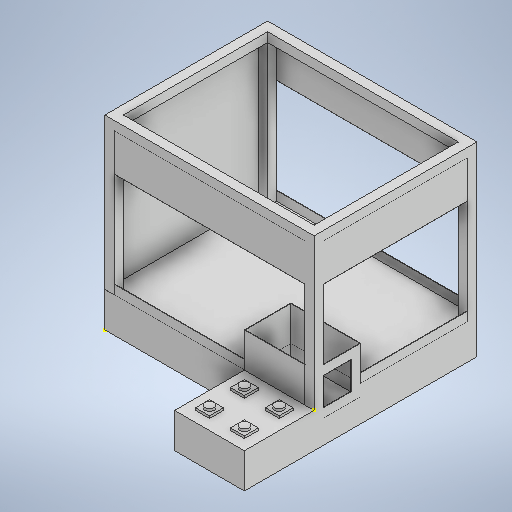
# Autodesk Inventor part: Project frame
Saved by Autodesk Inventor 2025.2 (Build 292293000, 293)
## iProperties
Created: 2025-01-26
Part Number: Project frame
Material: Generic
Document SubType Name: Modeling
Designer: Asus
Density: 1 g/cm^3
Appearance: Default
Author: Asus
Autodesk Inventor part; units mm, degrees
ref_plane "YZ Plane" through (0, 0, 0) normal (1, 0, 0) x (0, 1, 0)
ref_plane "XZ Plane" through (0, 0, 0) normal (0, 1, 0) x (-1, 0, 0)
ref_plane "XY Plane" through (0, 0, 0) normal (0, 0, 1) x (1, 0, 0)
sketch "Sketch1" plane through (0, 0, 0) normal (0, 1, 0) x (-1, 0, 0)
  line L0 (0, 0) -> (0, -350)
  line L1 (0, -350) -> (450, -350)
  line L2 (450, -350) -> (450, 0)
  line L3 (450, 0) -> (0, 0)
  dimension "d0" = 350
  dimension "d1" = 450
  constraints: 8 end point, 2 vertical, 1 horizontal, 1 perpendicular
  measures "d0" distance of L0.start L0.end
  measures "d1" distance of L0.end L1.end
extrude "Extrusion1" add sketch "Sketch1" along normal blind 75
sketch "Sketch2" plane through (0, 75, 0) normal (0, 1, 0) x (1, 0, 0)
  line L0 (-20, 350) -> (-20, 330)
  line L1 (-20, 330) -> (0, 330)
  line L2 (0, 350) -> (-450, 350) projected
  line L3 (0, 330) -> (0, 350)
  line L4 (0, 350) -> (-20, 350)
  point P0 (0, 0)
  dimension "d4" = 20
  dimension "d5" = 20
  constraints: 8 end point, 2 perpendicular, 1 collinear, 1 vertical
  measures "d4" distance of L0.start L0.end
  measures "d5" distance of L0.end L1.end
extrude "Extrusion2" add sketch "Sketch2" along normal blind 325
sketch "Sketch3" plane through (0, 75, 0) normal (0, 1, 0) x (1, 0, 0)
  point P0 (0, 0)
sketch "Sketch4" plane through (0, 75, 0) normal (0, 1, 0) x (1, 0, 0)
  line L0 (-20, 350) -> (-20, 330) projected
  line L1 (-20, 350) -> (-20, 349)
  line L2 (-20, 349) -> (-450, 349)
  line L3 (-450, 349) -> (-450, 350)
  line L4 (-450, 350) -> (-20, 350)
  line L5 (-20, 350) -> (-20, 349)
  line L6 (0, 0) -> (0, 350) projected
  line L7 (-20, 349) -> (-20, 350)
  line L8 (-20, 350) -> (-20, 349)
  dimension "d9" = 430
  dimension "d10" = 1
  dimension "d11" = 430
  dimension "d12" = 1
  constraints: 14 end point, 2 collinear, 2 perpendicular, 1 parallel, 1 point on line
  measures "d9" distance of L1.end L2.end
  measures "d10" distance of L2.end L3.end
  measures "d11" distance of L3.end L0.start
  measures "d12" distance of L0.start L1.end
extrude "Extrusion3" add sketch "Sketch4" along normal blind 20
sketch "Sketch5" plane through (0, 75, 0) normal (0, 1, 0) x (1, 0, 0)
  line L0 (-450, 350) -> (-450, 0) projected
  line L1 (-450, 350) -> (-449, 350)
  line L2 (-20, 350) -> (-450, 350) projected
  line L3 (-449, 350) -> (-449, 0)
  line L4 (-450, 0) -> (0, 0) projected
  line L5 (-449, 0) -> (-450, 0)
  line L6 (-450, 0) -> (-450, 350)
  line L7 (-20, 349) -> (-450, 349) projected
  line L8 (-449, 349) -> (-449, 350)
  line L9 (-450, 350) -> (-449, 350)
  dimension "d15" = 1
  constraints: 12 end point, 4 point on line, 3 collinear, 1 horizontal, 1 vertical
  measures "d15" distance of L0.start L1.end
extrude "Extrusion4" add sketch "Sketch5" along normal blind 325 contours L7 L3 L4 L0
sketch "Sketch6" plane through (0, 95, 0) normal (0, 1, 0) x (1, 0, 0)
  line L0 (-449, 349) -> (-449, 0) projected
  line L1 (-449, 349) -> (-449, 350)
  line L2 (-20, 350) -> (-450, 350) projected
  line L3 (-450, 350) -> (-450, 0) projected
  line L4 (-449, 350) -> (-450, 350)
  line L5 (-450, 350) -> (-450, 349)
  line L6 (-450, 349) -> (-449, 349) projected
  line L7 (-450, 349) -> (-449, 349)
  line L8 (-449, 349) -> (-449, 350)
  point P0 (0, 0)
  constraints: 10 end point, 3 collinear, 1 perpendicular, 1 point on line, 1 vertical
extrude "Extrusion5" add sketch "Sketch6" along normal blind 305
sketch "Sketch7" plane through (0, 75, 0) normal (0, 1, 0) x (1, 0, 0)
  line L0 (0, 0) -> (0, 350) projected
  line L1 (0, 0) -> (0, 20)
  line L2 (0, 20) -> (-20, 20)
  line L3 (-20, 20) -> (-20, 0)
  line L4 (-20, 0) -> (0, 0)
  dimension "d20" = 20
  dimension "d21" = 20
  constraints: 8 end point, 3 perpendicular, 1 point on line
  measures "d20" distance of L0.start L1.end
  measures "d21" distance of L1.end L2.end
extrude "Extrusion6" add sketch "Sketch7" along normal blind 325
sketch "Sketch8" plane through (0, 75, 0) normal (0, 1, 0) x (1, 0, 0)
  line L0 (0, 20) -> (-20, 20) projected
  line L1 (0, 20) -> (0, 100)
  line L2 (0, 20) -> (0, 330) projected
  line L3 (0, 100) -> (-1, 100)
  line L4 (-1, 100) -> (-1, 20)
  line L5 (-1, 20) -> (0, 20)
  point P0 (0, 0)
  dimension "d24" = 80
  dimension "d25" = 1
  dimension "d26" = 80
  constraints: 8 end point, 2 point on line, 1 collinear, 1 horizontal
  measures "d24" distance of L0.start L1.end
  measures "d25" distance of L1.end L3.end
  measures "d26" distance of L3.end L4.end
extrude "Extrusion7" add sketch "Sketch8" along normal blind 75
sketch "Sketch9" plane through (0, 75, 0) normal (0, 1, 0) x (1, 0, 0)
  line L0 (-1, 100) -> (0, 100) projected
  line L1 (-1, 100) -> (-149, 100)
  line L2 (-149, 100) -> (-149, 99)
  line L3 (-149, 99) -> (-1, 99)
  line L4 (-1, 100) -> (-1, 20) projected
  line L5 (-1, 99) -> (-1, 100)
  point P0 (0, 0)
  dimension "d29" = 148
  dimension "d32" = 1
  dimension "d33" = 148
  constraints: 8 end point, 1 horizontal, 1 perpendicular, 1 vertical
  measures "d29" distance of L0.start L1.end
  measures "d32" distance of L1.end L2.end
  measures "d33" distance of L2.end L3.end
extrude "Extrusion8" add sketch "Sketch9" along normal blind 75
sketch "Sketch10" plane through (0, 75, 0) normal (0, 1, 0) x (1, 0, 0)
  line L0 (-149, 99) -> (-149, 100) projected
  line L1 (-149, 100) -> (-150, 100)
  line L2 (-150, 100) -> (-150, 0)
  line L3 (-150, 0) -> (-149, 0)
  line L4 (-449, 0) -> (-20, 0) projected
  line L5 (-149, 0) -> (-149, 100)
  point P0 (0, 0)
  dimension "d36" = 1
  dimension "d37" = 100
  dimension "d38" = 1
  dimension "d39" = 100
  constraints: 8 end point, 1 horizontal, 1 point on line, 1 vertical
  measures "d36" distance of L0.end L1.end
  measures "d37" distance of L1.end L2.end
  measures "d38" distance of L2.end L3.end
  measures "d39" distance of L3.end L0.end
extrude "Extrusion9" add sketch "Sketch10" along normal blind 75
sketch "Sketch11" plane through (0, 75, 0) normal (0, 1, 0) x (1, 0, 0)
  line L0 (-450, 0) -> (0, 0) projected
  line L1 (-149.0001, 0) -> (-20.0001, 0)
  line L2 (-20.0001, 0) -> (-20.0001, 1)
  line L3 (-20.0001, 1) -> (-149.0001, 1)
  line L4 (-149.0001, 1) -> (-149.0001, 0)
  dimension "d42" = 129
  dimension "d43" = 1
  dimension "d44" = 129
  constraints: 8 end point, 2 perpendicular, 2 point on line
  measures "d42" distance of L1.start L1.end
  measures "d43" distance of L1.end L2.end
  measures "d44" distance of L2.end L3.end
extrude "Extrusion10" add sketch "Sketch11" along normal blind 75
sketch "Sketch12" plane through (0, 75, 0) normal (0, 1, 0) x (1, 0, 0)
  point P0 (0, 0)
sketch "Sketch13" plane through (0, 75, 0) normal (0, 1, 0) x (1, 0, 0)
  line L0 (-149, 1) -> (-149, 99) projected
  line L1 (-1, 20) -> (-1, 99) projected
  line L2 (-149, 99) -> (-1, 99)
  line L3 (-1, 99) -> (-1, 20)
  line L4 (0, 20) -> (-20, 20) projected
  line L5 (-1, 20) -> (-20, 20)
  line L6 (-20, 20) -> (-20, 1)
  line L7 (-20, 0) -> (0, 0) projected
  line L8 (-20, 1) -> (-149, 1)
  line L9 (-149, 1) -> (-149, 99)
  constraints: 12 end point, 4 perpendicular, 1 collinear, 1 horizontal
extrude "Extrusion11" cut sketch "Sketch13" against normal blind 25
sketch "Sketch14" plane through (0, 75, 0) normal (0, 1, 0) x (1, 0, 0)
  line L0 (0, 100) -> (0, 330) projected
  line L1 (0, 330) -> (0, 100)
  line L2 (0, 100) -> (-1, 100)
  line L3 (-150, 100) -> (0, 100) projected
  line L4 (0, 100) -> (1, 100) construction
  line L5 (-1, 100) -> (-1, 330)
  line L6 (-1, 330) -> (0, 330)
  point P0 (0, 0)
  dimension "d49" = 1
  dimension "d50" = 180
  dimension "d51" = 230
  dimension "d52" = 90
  constraints: 10 end point, 2 collinear, 1 horizontal, 1 perpendicular, 1 vertical
  measures "d49" distance of L0.start L2.end
  measures "d50" angle of L2 L4
  measures "d51" distance of L2.end L5.end
  measures "d52" angle of L2 L5
extrude "Extrusion12" add sketch "Sketch14" along normal blind 20
sketch "Sketch15" plane through (0, 75, 0) normal (0, 1, 0) x (1, 0, 0)
  line L0 (-449, 0) -> (-449, 350) projected
  line L1 (-150, 100) -> (-150, 0) projected
  line L2 (-449, 0) -> (-150, 0)
  line L3 (-150, 0) -> (-150, 1)
  line L4 (-150, 1) -> (-449, 1)
  line L5 (-449, 1) -> (-449, 0)
  point P0 (0, 0)
  dimension "d55" = 1
  dimension "d56" = 90
  constraints: 8 end point, 4 perpendicular
  measures "d55" distance of L1.end L3.end
  measures "d56" angle of L3 L2
extrude "Extrusion13" add sketch "Sketch15" along normal blind 20
sketch "Sketch16" plane through (0, 400, 0) normal (0, 1, 0) x (1, 0, 0)
  line L0 (-450, 350) -> (-450, 0) projected
  line L1 (-449, 0) -> (-449, 350) projected
  line L2 (-450, 350) -> (-449, 350)
  line L3 (-449, 350) -> (-449, 330)
  line L4 (-449, 330) -> (-450, 330)
  line L5 (-450, 330) -> (-450, 350)
  point P0 (0, 0)
  dimension "d59" = 20
  dimension "d60" = 20
  constraints: 8 end point, 4 perpendicular
  measures "d59" distance of L1.end L3.end
  measures "d60" distance of L4.end L0.start
extrude "Extrusion14" cut sketch "Sketch16" against normal blind 325
sketch "Sketch17" plane through (-449, 75, -349) normal (-1, 0, 0) x (0, 0, 1)
  line L0 (-1, 0) -> (-1, 20) projected
  line L1 (-1, 20) -> (-1, 0)
  line L2 (-1, 0) -> (0, 0)
  line L3 (0, 0) -> (0, 20)
  line L4 (0, 20) -> (-1, 20)
  point P0 (349, -75)
  dimension "d63" = 1
  constraints: 8 end point, 3 perpendicular, 1 vertical
  measures "d63" distance of L1.end L2.end
extrude "Extrusion15" cut sketch "Sketch17" against normal blind 19
sketch "Sketch18" plane through (0, 75, 0) normal (0, 1, 0) x (1, 0, 0)
  line L0 (-450, 350) -> (-430, 350) projected
  line L1 (-450, 350) -> (-430, 350)
  line L2 (-430, 350) -> (-430, 330)
  line L3 (-430, 330) -> (-450, 330)
  line L4 (-450, 330) -> (-450, 350)
  point P0 (0, 0)
  dimension "d66" = 20
  constraints: 8 end point, 3 perpendicular, 1 horizontal
  measures "d66" distance of L0.end L2.end
extrude "Extrusion16" add sketch "Sketch18" along normal blind 325
sketch "Sketch19" plane through (0, 400, 0) normal (0, 1, 0) x (1, 0, 0)
  line L0 (-449, 0) -> (-449, 1) projected
  line L1 (-450, 0) -> (0, 0) projected
  line L2 (-449, 0) -> (-450, 0)
  line L3 (-450, 0) -> (-450, 20)
  line L4 (-450, 20) -> (-449, 20)
  line L5 (-449, 20) -> (-449, 0)
  dimension "d69" = 20
  constraints: 8 end point, 2 perpendicular, 1 horizontal, 1 parallel
  measures "d69" distance of L1.start L3.end
extrude "Extrusion17" cut sketch "Sketch19" against normal blind 325
sketch "Sketch20" plane through (-449, 75, -1) normal (-1, 0, 0) x (0, 0, 1)
  line L0 (0, 19.9976) -> (1, 19.9976)
  line L1 (1, 19.9976) -> (1, -0.0024)
  line L2 (1, -0.0024) -> (0, -0.0024)
  line L3 (0, 19.9976) -> (0, -0.0024)
  point P0 (1, -75)
  dimension "d72" = 20
  constraints: 8 end point, 3 perpendicular, 1 horizontal
  measures "d72" distance of L0.end L1.end
extrude "Extrusion18" cut sketch "Sketch20" against normal blind 19
sketch "Sketch21" plane through (0, 95, 0) normal (0, 1, 0) x (1, 0, 0)
  line L0 (-150, 1) -> (-449, 1) projected
  line L1 (-449, 1) -> (-449, 0)
  line L2 (-449, 0) -> (-430, 0)
  line L3 (-430, 0) -> (-430, 1)
  line L4 (-430, 1) -> (-449, 1)
  point P0 (0, 0)
  dimension "d75" = 1
  dimension "d76" = 19
  dimension "d77" = 1
  constraints: 8 end point, 1 perpendicular, 1 point on line, 1 vertical
  measures "d75" distance of L0.end L1.end
  measures "d76" distance of L1.end L2.end
  measures "d77" distance of L2.end L3.end
extrude "Extrusion19" cut sketch "Sketch21" against normal blind 0.1
sketch "Sketch22" plane through (0, 75, 0) normal (0, 1, 0) x (1, 0, 0)
  line L0 (-450, 350) -> (-450, 0) projected
  line L1 (-450, 0) -> (-450, 20)
  line L2 (-450, 20) -> (-430, 20)
  line L3 (-430, 20) -> (-430, 0)
  line L4 (-430, 0) -> (-450, 0)
  point P0 (0, 0)
  dimension "d80" = 20
  dimension "d81" = 20
  constraints: 8 end point, 3 perpendicular, 1 point on line
  measures "d80" distance of L0.end L1.end
  measures "d81" distance of L1.end L2.end
extrude "Extrusion20" add sketch "Sketch22" along normal blind 325
sketch "Sketch23" plane through (-450, 0, 0) normal (0, 0, 1) x (1, 0, 0)
  line L0 (20, 75) -> (300, 75) projected
  line L1 (300, 75) -> (450, 75)
  line L2 (450, 0) -> (450, 400) projected
  line L3 (450, 75) -> (450, 0)
  line L4 (449, 150) -> (449, 50) projected
  line L5 (0, 0) -> (450, 0) projected
  line L6 (450, 0) -> (300, 0)
  line L7 (300, 75) -> (300, 0)
  constraints: 8 end point, 2 point on line, 1 horizontal, 1 parallel, 1 perpendicular
extrude "Extrusion21" add sketch "Sketch23" along normal blind 150
sketch "Sketch24" plane through (0, 75, 0) normal (0, 1, 0) x (1, 0, 0)
  line L0 (0, 0) -> (0, -150) projected
  line L1 (0, -75) -> (-150, -75)
  line L2 (-150, 0) -> (-150, -150) projected
  line L3 (0, -150) -> (-150, -150) projected
  line L4 (-75, -150) -> (-75, 0)
  line L5 (-127.5, -22.5) -> (-97.5, -22.5)
  line L6 (-97.5, -22.5) -> (-97.5, -52.5)
  line L7 (-97.5, -52.5) -> (-127.5, -52.5)
  line L8 (-127.5, -52.5) -> (-127.5, -22.5)
  line L9 (-127.5, -22.5) -> (-97.5, -52.5) construction
  line L10 (-97.5, -22.5) -> (-127.5, -52.5) construction
  line L11 (-52.5, -52.5) -> (-22.5, -52.5)
  line L12 (-22.5, -52.5) -> (-22.5, -22.5)
  line L13 (-22.5, -22.5) -> (-52.5, -22.5)
  line L14 (-52.5, -22.5) -> (-52.5, -52.5)
  line L15 (-52.5, -52.5) -> (-22.5, -22.5) construction
  line L16 (-22.5, -52.5) -> (-52.5, -22.5) construction
  line L17 (-52.5, -127.5) -> (-22.5, -127.5)
  line L18 (-22.5, -127.5) -> (-22.5, -97.5)
  line L19 (-22.5, -97.5) -> (-52.5, -97.5)
  line L20 (-52.5, -97.5) -> (-52.5, -127.5)
  line L21 (-52.5, -127.5) -> (-22.5, -97.5) construction
  line L22 (-22.5, -127.5) -> (-52.5, -97.5) construction
  line L23 (-127.5, -127.5) -> (-97.5, -127.5)
  line L24 (-97.5, -127.5) -> (-97.5, -97.5)
  line L25 (-97.5, -97.5) -> (-127.5, -97.5)
  line L26 (-127.5, -97.5) -> (-127.5, -127.5)
  line L27 (-127.5, -127.5) -> (-97.5, -97.5) construction
  line L28 (-97.5, -127.5) -> (-127.5, -97.5) construction
  dimension "d86" = 30
  dimension "d87" = 30
  dimension "d88" = 30
  constraints: 52 end point, 8 parallel, 4 horizontal, 4 perpendicular, 4 point on line, 3 midpoint, 1 vertical
  measures "d86" distance of L6.end L7.end
  measures "d87" distance of L5.end L6.end
  measures "d88" distance of L13.end L12.end
extrude "Extrusion22" add sketch "Sketch24" along normal blind 5 contours L5 L6 L7 L8 | L14 L13 L12 L11 | L20 L19 L18 L17 | L26 L25 L24 L23
sketch "Sketch25" plane through (0, 75, 0) normal (0, 1, 0) x (1, 0, 0)
  circle A0 centre (-37.5, -112.5) radius 10
  point P0 (0, 0)
  dimension "d91" = 20
  constraints: 1 centre point
  measures "d91" diameter of A0
extrude "Extrusion23" add sketch "Sketch25" along normal blind 10
sketch "Sketch26" plane through (0, 80, 0) normal (0, 1, 0) x (1, 0, 0)
  circle A0 centre (-112.5, -112.5) radius 10
  point P0 (0, 0)
  dimension "d94" = 20
  constraints: 1 centre point
  measures "d94" diameter of A0
extrude "Extrusion24" add sketch "Sketch26" along normal blind 5
sketch "Sketch27" plane through (0, 80, 0) normal (0, 1, 0) x (1, 0, 0)
  circle A0 centre (-112.5, -37.5) radius 10
  point P0 (0, 0)
  dimension "d97" = 20
  constraints: 1 centre point
  measures "d97" diameter of A0
extrude "Extrusion25" add sketch "Sketch27" along normal blind 5
sketch "Sketch28" plane through (0, 80, 0) normal (0, 1, 0) x (1, 0, 0)
  circle A0 centre (-37.5, -37.5) radius 10
  point P0 (0, 0)
  dimension "d100" = 20
  constraints: 1 centre point
  measures "d100" diameter of A0
extrude "Extrusion26" add sketch "Sketch28" along normal blind 5
sketch "Sketch29" plane through (0, 0, -350) normal (0, 0, -1) x (-1, 0, 0)
  line L0 (20, 75) -> (20, 400) projected
  line L1 (430, 95) -> (430, 400) projected
  line L2 (20, 400) -> (430, 400)
  line L3 (430, 400) -> (430, 380)
  line L4 (430, 380) -> (20, 380)
  line L5 (20, 380) -> (20, 400)
  point P0 (0, 0)
  dimension "d103" = 20
  constraints: 8 end point, 1 horizontal, 1 parallel, 1 perpendicular, 1 point on line
  measures "d103" distance of L1.end L3.end
extrude "Extrusion27" add sketch "Sketch29" against normal blind 20
sketch "Sketch30" plane through (-450, 0, 0) normal (0, 0, 1) x (1, 0, 0)
  line L0 (20, 380) -> (430, 380) projected
  line L1 (430, 75) -> (430, 380) projected
  line L2 (20, 380) -> (430, 380)
  line L3 (430, 380) -> (430, 400)
  line L4 (430, 400) -> (20, 400)
  line L5 (20, 400) -> (20, 380)
  point P0 (450, 0)
  dimension "d106" = 20
  dimension "d107" = 20
  constraints: 8 end point, 3 perpendicular, 1 collinear
  measures "d106" distance of L0.end L3.end
  measures "d107" distance of L4.end L0.start
extrude "Extrusion28" add sketch "Sketch30" against normal blind 20
sketch "Sketch31" plane through (0, 0, -350) normal (1, 0, 0) x (0, 0, -1)
  line L0 (-330, 400) -> (-330, 75) projected
  line L1 (-20, 95) -> (-20, 400) projected
  line L2 (-330, 400) -> (-20, 400)
  line L3 (0, 380) -> (-20, 380) projected
  line L4 (-20, 400) -> (-20, 380)
  line L5 (-20, 380) -> (-330, 380)
  line L6 (-350, 0) -> (-350, 400) projected
  line L7 (-330, 380) -> (-330, 400)
  dimension "d110" = 20
  constraints: 8 end point, 4 perpendicular
  measures "d110" distance of L5.end L0.start
extrude "Extrusion29" add sketch "Sketch31" against normal blind 20
sketch "Sketch32" plane through (0, 400, 0) normal (0, 1, 0) x (1, 0, 0)
  line L0 (-449, 20) -> (-430, 20) projected
  line L1 (-449, 20) -> (-450, 20)
  line L2 (-450, 350) -> (-450, 0) projected
  line L3 (-449, 20) -> (-449, 330) projected
  line L4 (-449, 330) -> (-450, 330)
  point P0 (0, 0)
  constraints: 4 end point, 2 horizontal, 1 point on line
extrude "Extrusion30" cut sketch "Sketch32" against normal blind 20
sketch "Sketch33" plane through (-450, 0, -350) normal (-1, 0, 0) x (0, 0, 1)
  point P0 (350, 0)
sketch "Sketch34" plane through (-450, 0, -350) normal (-1, 0, 0) x (0, 0, 1)
  line L0 (330, 380) -> (20, 380) projected
  line L1 (20, 380) -> (20, 400)
  line L2 (20, 400) -> (330, 400)
  line L3 (330, 400) -> (330, 380)
  line L4 (20, 380) -> (330, 380)
  point P0 (350, 0)
  dimension "d115" = 20
  constraints: 8 end point, 2 equal length, 1 perpendicular, 1 vertical
  measures "d115" distance of L0.end L1.end
extrude "Extrusion31" add sketch "Sketch34" against normal blind 20
sketch "Sketch35" plane through (0, 0, -350) normal (0, 0, -1) x (-1, 0, 0)
  line L0 (20, 380) -> (430, 380) projected
  line L1 (20, 380) -> (20, 300)
  line L2 (20, 75) -> (20, 380) projected
  line L3 (20, 300) -> (430, 300)
  line L4 (430, 75) -> (430, 380) projected
  point P0 (0, 0)
  dimension "d118" = 80
  constraints: 4 end point, 2 point on line, 1 perpendicular
  measures "d118" distance of L0.start L1.end
extrude "Extrusion32" add sketch "Sketch35" against normal blind 1
sketch "Sketch36" plane through (0, 0, -350) normal (1, 0, 0) x (0, 0, -1)
  line L0 (-330, 380) -> (-20, 380) projected
  line L1 (-20, 380) -> (-20, 300)
  line L2 (-20, 75) -> (-20, 380) projected
  line L3 (-20, 300) -> (-330, 300)
  line L4 (-330, 380) -> (-330, 75) projected
  point P0 (-350, 0)
  dimension "d121" = 80
  constraints: 4 end point, 2 point on line, 1 perpendicular
  measures "d121" distance of L0.end L1.end
extrude "Extrusion33" add sketch "Sketch36" against normal blind 1
sketch "Sketch37" plane through (-450, 400, 0) normal (0, 0, 1) x (1, 0, 0)
  line L0 (20, -20) -> (1, -20) projected
  line L1 (430, -100) -> (20, -100) projected
  line L2 (20, -20) -> (20, -100)
  line L3 (20, -100) -> (430, -100)
  line L4 (430, -100) -> (430, -20)
  line L5 (430, -20) -> (20, -20)
  point P0 (450, -400)
  dimension "d124" = 80
  dimension "d125" = 410
  dimension "d126" = 80
  dimension "d127" = 410
  constraints: 8 end point, 3 perpendicular
  measures "d124" distance of L0.start L1.end
  measures "d125" distance of L1.end L1.start
  measures "d126" distance of L1.start L4.end
  measures "d127" distance of L4.end L0.start
extrude "Extrusion34" add sketch "Sketch37" against normal blind 1
sketch "Sketch38" plane through (0, 0, -350) normal (1, 0, 0) x (0, 0, -1)
  line L0 (-330, 130) -> (-270, 130)
  line L1 (-270, 130) -> (-270, 70)
  line L2 (-270, 70) -> (-330, 70)
  line L3 (-330, 70) -> (-330, 130)
  point P0 (-350, 0)
  point P1 (-330, 150)
  dimension "d131" = 60
  dimension "d132" = 60
  dimension "d133" = 60
  constraints: 8 end point, 1 horizontal, 1 vertical
  measures "d131" distance of L0.start L0.end
  measures "d132" distance of L0.end L1.end
  measures "d133" distance of L1.end L2.end
extrude "Extrusion35" cut sketch "Sketch38" against normal blind 1
body "Solid1"
